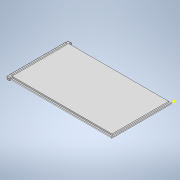
# Autodesk Inventor part: Case-Top
Saved by Autodesk Inventor 2020.2 (Build 242310000, 310)
## iProperties
Created: 2020-03-07
Part Number: Case-Top
Material: Generic
Document SubType Name: Modeling
Designer: dnguy
Density: 1 g/cm^3
Appearance: Default
Author: dnguy
Autodesk Inventor part; units mm, degrees
ref_plane "YZ Plane" through (0, 0, 0) normal (1, 0, 0) x (0, 1, 0)
ref_plane "XZ Plane" through (0, 0, 0) normal (0, 1, 0) x (-1, 0, 0)
ref_plane "XY Plane" through (0, 0, 0) normal (0, 0, 1) x (1, 0, 0)
ref_plane "Work Plane5" through (-116, 33, 0) normal (-1, 0, 0) x (0, 0, 1)
sketch "Sketch3" plane through (-116, 33, 0) normal (-1, 0, 0) x (0, 0, 1)
  line L0 (0, 0) -> (0, 3) projected
  line L1 (70, -31) -> (70, 0) projected
  line L2 (0, 3) -> (70, 3)
  line L3 (70, 3) -> (70, 0)
  line L4 (70, 0) -> (0, 0)
  line L5 (0, 0) -> (0, 3)
  point P0 (0, -33)
  constraints: 8 end point, 2 parallel, 1 horizontal, 1 perpendicular
extrude "Extrusion1" add sketch "Sketch3" along normal blind 3.8
ref_plane "Work Plane6" through (-116, 33, 0) normal (1, 0, 0) x (0, 0, -1)
sketch "Sketch4" plane through (-116, 33, 0) normal (1, 0, 0) x (0, 0, -1)
  line L0 (-3, 0) -> (-67, 0) projected
  line L1 (-67, 0) -> (-35, 0)
  line L2 (-67, 3) -> (-3, 3) projected
  line L3 (-67, 0) -> (-35, 0) construction
  line L4 (-35, 0) -> (-35, 0.75)
  line L5 (-68.5, 0.75) -> (-1.5, 0.75) construction
  line L6 (-15, 0) -> (-55, 0) projected
  line L7 (-68.5, 0.1) -> (-1.5, 0.1)
  line L8 (-1.5, 1.4) -> (-68.5, 1.4)
  arc A0 (-68.5, 1.4) -> (-68.5, 0.1) centre (-68.5, 0.75) ccw
  arc A1 (-1.5, 0.1) -> (-1.5, 1.4) centre (-1.5, 0.75) ccw
  line L9 (-35, 0.75) -> (32, 0.75) construction
  point P0 (0, -33)
  dimension "d3" = 32
  dimension "d4" = 0
  dimension "d5" = 0.75
  dimension "d6" = 33.5
  dimension "d7" = 0
  dimension "d8" = 1.3
  constraints: 16 end point, 4 point on circle, 4 tangent, 3 parallel, 2 centre point, 2 collinear, 2 horizontal, 1 midpoint, 1 perpendicular
  measures "d3" distance of L0.end L1.end
  measures "d4" distance between parallel lines of L1 L3
  measures "d5" distance of L1.end L4.end
  measures "d6" distance of L4.end L5.end
  measures "d7" distance between parallel lines of L5 L9
  measures "d8" diameter of A1
extrude "Extrusion2" add sketch "Sketch4" along normal blind 114.3
ref_plane "Work Plane7" through (-116, 34.4, 68.5) normal (0, 1, 0) x (1, 0, 0)
sketch "Sketch5" plane through (-116, 34.4, 68.5) normal (0, 1, 0) x (1, 0, 0)
  line L0 (113, 1.5) -> (0, 1.5) projected
  line L1 (0, 65.5) -> (0, 1.5) projected
  line L2 (113, 1.5) -> (0, 1.5)
  line L3 (0, 1.5) -> (0, 65.5)
  line L4 (0, 65.5) -> (113, 65.5)
  line L5 (113, 65.5) -> (113, 1.5)
  point P0 (116, 68.5)
  constraints: 8 end point, 2 parallel, 1 horizontal, 1 perpendicular
extrude "Extrusion3" add sketch "Sketch5" along normal blind 1.6
sketch "Sketch6" plane through (-116, 33, 0) normal (0, -1, 0) x (1, 0, 0)
  line L0 (0, 70) -> (-3.8, 70) projected
  line L1 (-1.9, 70) -> (-1.9, 35.5)
  line L2 (-3.8, 70) -> (-3.8, 0) projected
  line L3 (-1.9, 70) -> (32.6, 70) construction
  line L4 (-1.9, 16) -> (-1.9, 55) construction
  line L5 (-1.275, 16) -> (-1.275, 55)
  line L6 (-2.525, 55) -> (-2.525, 16)
  arc A0 (-2.525, 16) -> (-1.275, 16) centre (-1.9, 16) ccw
  arc A1 (-1.275, 55) -> (-2.525, 55) centre (-1.9, 55) ccw
  line L7 (-1.9, 35.5) -> (37.1, 35.5) construction
  point P0 (116, 0)
  dimension "d14" = 34.5
  dimension "d15" = 90
  dimension "d16" = 19.5
  dimension "d17" = 90
  dimension "d18" = 1.25
  constraints: 14 end point, 4 point on circle, 4 tangent, 2 centre point, 2 horizontal, 2 midpoint, 2 parallel, 2 perpendicular, 1 collinear
  measures "d14" distance of L1.start L1.end
  measures "d15" angle of L1 L3
  measures "d16" distance of L1.end L4.end
  measures "d17" angle of L7 L4
  measures "d18" diameter of A1
extrude "Extrusion4" add sketch "Sketch6" along normal blind 0.95 draft -65
sketch "Sketch7" plane through (-119.8, 36, 70) normal (0, 1, 0) x (1, 0, 0)
  line L0 (116.8, 67) -> (3.8, 67) projected
  line L1 (3.8, 67) -> (3.8, 35)
  line L2 (3.8, 3) -> (116.8, 3) projected
  line L3 (3.8, 35) -> (2.05, 35)
  line L4 (2.525, 15) -> (2.525, 54) projected
  line L5 (3.8, 35) -> (5.55, 35) construction
  line L6 (2.05, 65) -> (2.05, 5) construction
  line L7 (1.9, 54) -> (1.9, 15) projected
  line L8 (1.3, 65) -> (1.3, 5)
  line L9 (2.8, 5) -> (2.8, 65)
  arc A0 (2.8, 65) -> (1.3, 65) centre (2.05, 65) ccw
  arc A1 (1.3, 5) -> (2.8, 5) centre (2.05, 5) ccw
  line L10 (2.05, 35) -> (62.05, 35) construction
  point P0 (119.8, 70)
  dimension "d21" = 32
  dimension "d32" = 1.75
  dimension "d33" = 180
  dimension "d34" = 30
  dimension "d35" = 90
  dimension "d36" = 1.5
  constraints: 12 end point, 4 point on circle, 4 tangent, 3 horizontal, 2 centre point, 2 perpendicular, 1 collinear, 1 parallel, 7 other
  measures "d21" distance of L0.end L1.end
  measures "d32" distance of L1.end L3.end
  measures "d33" angle of L3 L5
  measures "d34" distance of L3.end A1.centre
  measures "d35" angle to the sketch y axis of L10
  measures "d36" diameter of A1
extrude "Extrusion5" add sketch "Sketch7" along normal blind 0.5
fillet "Fillet2" radius 1 4 edges at (-117.75, 36, 4.25) (-117, 36, 35) (-117.75, 36, 65.75) (-118.5, 36, 35)
sketch "Sketch8" plane through (-119.8, 36, 70) normal (0, 1, 0) x (1, 0, 0)
  point P0 (119.8, 70)
fillet "Fillet3" radius 1 1 edges at (-119.8, 36, 35)
fillet "Fillet4" radius 1 6 edges at (-119.5071, 35.7071, 0) (-119.8, 34, 0) (-117.4, 36, 0) (-119.5071, 35.7071, 70) (-119.8, 34, 70) (-117.4, 36, 70)
body "Solid1"
